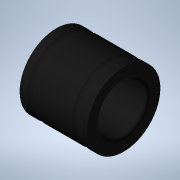
# Autodesk Inventor part: 2200 Inner Ring
Saved by Autodesk Inventor 2021 (Build 250183000, 183)
## iProperties
Created: 2026-07-02
Part Number: 2200 Inner Ring
Material: Generic
Catalog Web Link: www.3dfindit.com
Description: cylindrical_bore_IR-
Vendor: NSK_RB
Document SubType Name: Modeling
Designer: psAdmin
Manufacturer: NSK_RB
Mass: 1.42261 g
Surface Area: 12.9944 cm^2
Volume: 1.42261 cm^3
Density: 1 g/cm^3
Appearance: PSOLRGB-128-128-128
Category: PARTsolutions
Company: NSK_RB
Title: 2200 Inner Ring
Author: Cadenas PARTsolutions
PSOL_IDENT_0: {$CADENAS_DATA/23d-libs/nsk_rb/roller_bearings/self_aliging_bb/cylindrical_bore_ir.prj},184 {VTYP=3D
PSOL_IDENT_1: },{NB=2200 Inner Ring},{LINA=2200 Inner Ring},{NN=cylindrical_bore_IR},{DATE=06.08.2025 00:27:17},{G
PSOL_IDENT_2: EOMDATE=17.08.2022 06:34:33},{VERSION=},{LINEID=120},{WBVAR=},{WBNUMERIC=}  {NB=2200 Inner Ring},{LI
PSOL_IDENT_3: NA=2200 Inner Ring},{KT=DUMMY},{IDNR=},{STAN=},{ORDER=2200},{SD=10},{X=10},{D=30},{DD=30},{B=14},{R=
PSOL_IDENT_4: 0.6},{SDE1=22.420},{DI1=15.20},{CR1=7450},{COR1=1590},{CR2=760},{COR2=162},{LG=24000},{LO=28000},{DA
PSOL_IDENT_5: 1=14.0},{DA2=26.0},{RA=0.6},{E=0.64},{Y2=1.5},{Y3=0.98},{Y0=1.00},{MASS=0.042},{SC=1},{N=8},{DIST=1.
PSOL_IDENT_6: 467}
NB: 2200 Inner Ring
NN: cylindrical_bore_IR
NBSYN: $ORDER. Inner Ring
LINA: 2200 Inner Ring
CATALOG: NSK Rolling Bearing
ORDER: 2200
SD: 10
X: 10
D: 30
DD: 30
B: 14
R: 0.6
SDE1: 22.42
DI1: 15.2
CR1: 7450
COR1: 1590
CR2: 760
COR2: 162
LG: 24000
LO: 28000
DA1: 14
DA2: 26
RA: 0.6
E: 0.64
Y2: 1.5
Y3: 0.98
Y0: 1
MASS: 0.042
SC: 1
SUPPLIER: NSK_RB
ARTICLENO: 2200 Inner Ring
BOMINFO: 2200 Inner Ring
CREATOR: CADENAS GmbH
Autodesk Inventor part; units mm, degrees
sketch "Sketch_1" plane through (0, 0, 0) normal (0, 0, 1) x (1, 0, 0)
  line L0 (14, 0) -> (0, 0)
  arc A0 (0, 5.6) -> (0.6, 5) centre (0.6, 5.6) ccw
  line L1 (0.6, 5) -> (13.4, 5)
  arc A1 (13.4, 5) -> (14, 5.6) centre (13.4, 5.6) ccw
  line L2 (14, 5.6) -> (14, 7.6)
  line L3 (14, 7.6) -> (12.4286, 7.6)
  arc A2 (10.8662, 7.6) -> (12.4286, 7.6) centre (11.6474, 9.8192) ccw
  line L4 (10.8662, 7.6) -> (3.1338, 7.6)
  arc A3 (1.5714, 7.6) -> (3.1338, 7.6) centre (2.3526, 9.8192) ccw
  line L5 (1.5714, 7.6) -> (0, 7.6)
  line L6 (0, 7.6) -> (0, 5.6)
  constraints: 14 end point, 8 point on circle, 4 centre point
revolve "Revolution1" add sketch "Sketch_1" angle 360 about axis through (14, 0, 0) along (1, 0, 0)
ref_plane "ip_cb_11_1_XY" through (2.3526, 9.0717, 3.7576) normal (1, 0, 0) x (0, 0, -1)
ref_plane "ip_cb_11_1_YZ" through (2.3526, 9.0717, 3.7576) normal (0, 0, -1) x (0, 1, 0)
ref_plane "ip_cb_11_1_ZX" through (2.3526, 9.0717, 3.7576) normal (0, 1, 0) x (1, 0, 0)
ref_plane "ip_cb_11_2_XY" through (2.3526, 3.7576, 9.0717) normal (1, 0, 0) x (0, 0, -1)
ref_plane "ip_cb_11_2_YZ" through (2.3526, 3.7576, 9.0717) normal (0, 0, -1) x (0, 1, 0)
ref_plane "ip_cb_11_2_ZX" through (2.3526, 3.7576, 9.0717) normal (0, 1, 0) x (1, 0, 0)
ref_plane "ip_cb_11_3_XY" through (2.3526, -3.7576, 9.0717) normal (1, 0, 0) x (0, 0, -1)
ref_plane "ip_cb_11_3_YZ" through (2.3526, -3.7576, 9.0717) normal (0, 0, -1) x (0, 1, 0)
ref_plane "ip_cb_11_3_ZX" through (2.3526, -3.7576, 9.0717) normal (0, 1, 0) x (1, 0, 0)
ref_plane "ip_cb_11_4_XY" through (2.3526, -9.0717, 3.7576) normal (1, 0, 0) x (0, 0, -1)
ref_plane "ip_cb_11_4_YZ" through (2.3526, -9.0717, 3.7576) normal (0, 0, -1) x (0, 1, 0)
ref_plane "ip_cb_11_4_ZX" through (2.3526, -9.0717, 3.7576) normal (0, 1, 0) x (1, 0, 0)
ref_plane "ip_cb_11_5_XY" through (2.3526, -9.0717, -3.7576) normal (1, 0, 0) x (0, 0, -1)
ref_plane "ip_cb_11_5_YZ" through (2.3526, -9.0717, -3.7576) normal (0, 0, -1) x (0, 1, 0)
ref_plane "ip_cb_11_5_ZX" through (2.3526, -9.0717, -3.7576) normal (0, 1, 0) x (1, 0, 0)
ref_plane "ip_cb_11_6_XY" through (2.3526, -3.7576, -9.0717) normal (1, 0, 0) x (0, 0, -1)
ref_plane "ip_cb_11_6_YZ" through (2.3526, -3.7576, -9.0717) normal (0, 0, -1) x (0, 1, 0)
ref_plane "ip_cb_11_6_ZX" through (2.3526, -3.7576, -9.0717) normal (0, 1, 0) x (1, 0, 0)
ref_plane "ip_cb_11_7_XY" through (2.3526, 3.7576, -9.0717) normal (1, 0, 0) x (0, 0, -1)
ref_plane "ip_cb_11_7_YZ" through (2.3526, 3.7576, -9.0717) normal (0, 0, -1) x (0, 1, 0)
ref_plane "ip_cb_11_7_ZX" through (2.3526, 3.7576, -9.0717) normal (0, 1, 0) x (1, 0, 0)
ref_plane "ip_cb_11_8_XY" through (2.3526, 9.0717, -3.7576) normal (1, 0, 0) x (0, 0, -1)
ref_plane "ip_cb_11_8_YZ" through (2.3526, 9.0717, -3.7576) normal (0, 0, -1) x (0, 1, 0)
ref_plane "ip_cb_11_8_ZX" through (2.3526, 9.0717, -3.7576) normal (0, 1, 0) x (1, 0, 0)
ref_plane "ip_cb_1a_XY" through (0, 0, 0) normal (-1, 0, 0) x (0, 0, -1)
ref_plane "ip_cb_1a_YZ" through (0, 0, 0) normal (0, 0, -1) x (0, -1, 0)
ref_plane "ip_cb_1a_ZX" through (0, 0, 0) normal (0, -1, 0) x (-1, 0, 0)
ref_plane "ip_cb_22_1_XY" through (11.6474, 9.8192, 0) normal (1, 0, 0) x (0, 0, -1)
ref_plane "ip_cb_22_1_YZ" through (11.6474, 9.8192, 0) normal (0, 0, -1) x (0, 1, 0)
ref_plane "ip_cb_22_1_ZX" through (11.6474, 9.8192, 0) normal (0, 1, 0) x (1, 0, 0)
ref_plane "ip_cb_22_2_XY" through (11.6474, 6.9432, 6.9432) normal (1, 0, 0) x (0, 0, -1)
ref_plane "ip_cb_22_2_YZ" through (11.6474, 6.9432, 6.9432) normal (0, 0, -1) x (0, 1, 0)
ref_plane "ip_cb_22_2_ZX" through (11.6474, 6.9432, 6.9432) normal (0, 1, 0) x (1, 0, 0)
ref_plane "ip_cb_22_3_XY" through (11.6474, 0, 9.8192) normal (1, 0, 0) x (0, 0, -1)
ref_plane "ip_cb_22_3_YZ" through (11.6474, 0, 9.8192) normal (0, 0, -1) x (0, 1, 0)
ref_plane "ip_cb_22_3_ZX" through (11.6474, 0, 9.8192) normal (0, 1, 0) x (1, 0, 0)
ref_plane "ip_cb_22_4_XY" through (11.6474, -6.9432, 6.9432) normal (1, 0, 0) x (0, 0, -1)
ref_plane "ip_cb_22_4_YZ" through (11.6474, -6.9432, 6.9432) normal (0, 0, -1) x (0, 1, 0)
ref_plane "ip_cb_22_4_ZX" through (11.6474, -6.9432, 6.9432) normal (0, 1, 0) x (1, 0, 0)
ref_plane "ip_cb_22_5_XY" through (11.6474, -9.8192, 0) normal (1, 0, 0) x (0, 0, -1)
ref_plane "ip_cb_22_5_YZ" through (11.6474, -9.8192, 0) normal (0, 0, -1) x (0, 1, 0)
ref_plane "ip_cb_22_5_ZX" through (11.6474, -9.8192, 0) normal (0, 1, 0) x (1, 0, 0)
ref_plane "ip_cb_22_6_XY" through (11.6474, -6.9432, -6.9432) normal (1, 0, 0) x (0, 0, -1)
ref_plane "ip_cb_22_6_YZ" through (11.6474, -6.9432, -6.9432) normal (0, 0, -1) x (0, 1, 0)
ref_plane "ip_cb_22_6_ZX" through (11.6474, -6.9432, -6.9432) normal (0, 1, 0) x (1, 0, 0)
ref_plane "ip_cb_22_7_XY" through (11.6474, 0, -9.8192) normal (1, 0, 0) x (0, 0, -1)
ref_plane "ip_cb_22_7_YZ" through (11.6474, 0, -9.8192) normal (0, 0, -1) x (0, 1, 0)
ref_plane "ip_cb_22_7_ZX" through (11.6474, 0, -9.8192) normal (0, 1, 0) x (1, 0, 0)
ref_plane "ip_cb_22_8_XY" through (11.6474, 6.9432, -6.9432) normal (1, 0, 0) x (0, 0, -1)
ref_plane "ip_cb_22_8_YZ" through (11.6474, 6.9432, -6.9432) normal (0, 0, -1) x (0, 1, 0)
ref_plane "ip_cb_22_8_ZX" through (11.6474, 6.9432, -6.9432) normal (0, 1, 0) x (1, 0, 0)
body "Solid1"
